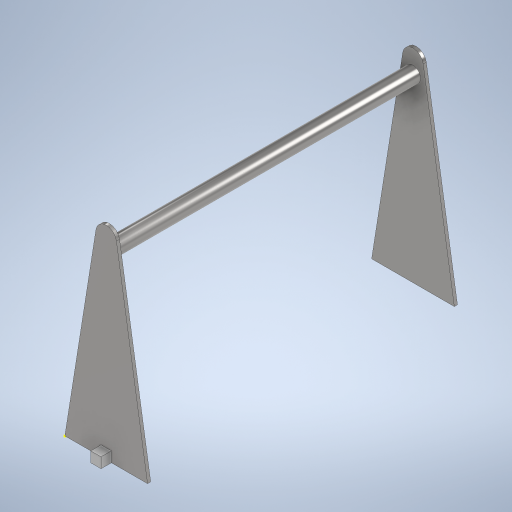
# Autodesk Inventor part: stand
Saved by Autodesk Inventor 2024 (Build 280153000, 153)
## iProperties
Created: 2024-01-19
Part Number: stand
Material: Generic
Document SubType Name: Modeling
Designer: HP
Density: 1 g/cm^3
Appearance: Default
Author: HP
Autodesk Inventor part; units mm, degrees
ref_plane "YZ Plane" through (0, 0, 0) normal (1, 0, 0) x (0, 1, 0)
ref_plane "XZ Plane" through (0, 0, 0) normal (0, 1, 0) x (-1, 0, 0)
ref_plane "XY Plane" through (0, 0, 0) normal (0, 0, 1) x (1, 0, 0)
sketch "Sketch1" plane through (0, 0, 0) normal (0, 0, 1) x (1, 0, 0)
  point P0 (0, 0)
sketch "Sketch2" plane through (0, 0, 0) normal (0, 0, 1) x (1, 0, 0)
  line L0 (0, 0) -> (80, 0)
  line L1 (80, 0) -> (40, 250)
  line L2 (40, 250) -> (0, 0)
  dimension "d0" = 80
  dimension "d1" = 250
  dimension "d2" = 40
  constraints: 6 end point, 1 horizontal
  measures "d0" distance of L0.start L0.end
  measures "d1" distance from line of L0 L1.end
  measures "d2" horizontal distance of L0.start L1.end
extrude "Extrusion1" add sketch "Sketch2" against normal blind 3
sketch "Sketch3" plane through (0, 0, -3) normal (0, 0, -1) x (-1, 0, 0)
  circle A0 centre (-40, 175) radius 7.5
  line L0 (-80, 0) -> (0, 0) projected
  point P0 (-40, 250)
  point P1 (-40, 0)
  dimension "d5" = 15
  dimension "d6" = 0
  dimension "d7" = 175
  constraints: 1 centre point, 1 midpoint
  measures "d5" diameter of A0
  measures "d6" horizontal distance of point (-40, 250) A0.centre
  measures "d7" distance of point (-40, 0) A0.centre
fillet "Fillet1" radius 10 1 edges at (40, 250, -1.5)
extrude "Extrusion2" add sketch "Sketch3" along normal blind 147
mirror "Mirror1" about plane through (40, 175, -150) normal (0, 0, -1) of "Extrusion2", "Extrusion1"
fillet "Fillet2" radius 10 1 edges at (40, 250, -298.5)
sketch "Sketch8" plane through (0, 0, 0) normal (0, 0, 1) x (1, 0, 0)
  line L0 (0, 0) -> (80, 0) projected
  line L1 (35, 0) -> (45, 0)
  line L2 (45, 0) -> (45, 10)
  line L3 (45, 10) -> (35, 10)
  line L4 (35, 10) -> (35, 0)
  point P0 (40, 0)
  point P1 (40, 10)
  point P2 (35, 5)
  dimension "d30" = 10
  dimension "d31" = 10
  dimension "d32" = 35
  constraints: 8 end point, 3 midpoint, 2 parallel, 1 horizontal, 1 perpendicular, 1 point on line
  measures "d30" distance of L3.end L2.end
  measures "d31" distance of point (40, 0) point (40, 10)
  measures "d32" horizontal distance of L0.start point (35, 5)
extrude "Extrusion7" add sketch "Sketch8" along normal blind 10
body "Solid1"
